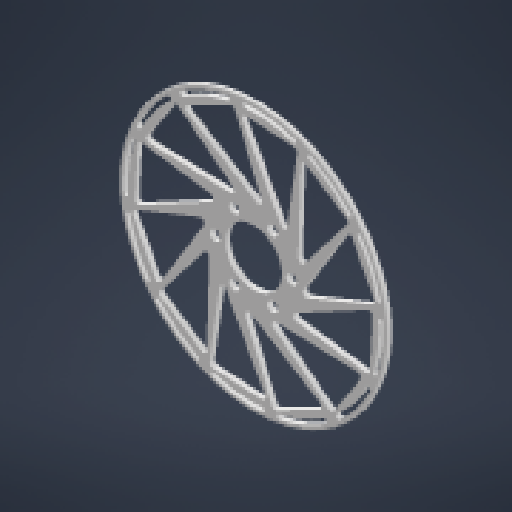
# Autodesk Inventor part: DisqueFrein
Saved by Autodesk Inventor 2026.2 (Build 302298010, 298A)
## iProperties
Created: 2026-04-18
Part Number: DisqueFrein
Material: Générique
Document SubType Name: Modeling
Designer: romai
Density: 1 g/cm^3
Appearance: Par défaut
Author: romai
Autodesk Inventor part; units mm, degrees
ref_plane "YZ Plane" through (0, 0, 0) normal (1, 0, 0) x (0, 1, 0)
ref_plane "XZ Plane" through (0, 0, 0) normal (0, 1, 0) x (-1, 0, 0)
ref_plane "XY Plane" through (0, 0, 0) normal (0, 0, 1) x (1, 0, 0)
sketch "Esquisse1" plane through (0, 0, 0) normal (0, 0, 1) x (1, 0, 0)
  circle A0 centre (0, 0) radius 16.25
  circle A1 centre (0, 0) radius 77.5
  line L0 (1.7183, 28.683) -> (-38.4934, 53.5132)
  line L1 (-10.6387, 68.5856) -> (4.6212, 31.1395)
  arc A2 (1.7183, 28.683) -> (4.6212, 31.1395) centre (2.7691, 30.3848) ccw
  arc A3 (-38.5051, 56.9093) -> (-38.4934, 53.5132) centre (-37.4426, 55.2149) ccw
  arc A4 (-10.6387, 68.5856) -> (-13.2718, 69.672) centre (-12.4908, 67.8308) ccw
  line L2 (-38.5051, 56.9093) -> (-13.2718, 69.672)
  arc A5 (-14.9639, 73.4921) -> (-41.9265, 62.1866) centre (0, 0) ccw
  arc A6 (-14.4371, 71.048) -> (-40.4825, 60.1449) centre (0, 0) ccw
  line L3 (-41.8018, 60.3256) -> (-42.1283, 60.7085)
  line L4 (-13.6695, 72.2839) -> (-13.7977, 72.768)
  arc A7 (-41.8018, 60.3256) -> (-40.4825, 60.1449) centre (-41.0409, 60.9745) ccw
  arc A8 (-41.9265, 62.1866) -> (-42.1283, 60.7085) centre (-41.3675, 61.3574) ccw
  arc A9 (-13.7977, 72.768) -> (-14.9639, 73.4921) centre (-14.7644, 72.5122) ccw
  arc A10 (-14.4371, 71.048) -> (-13.6695, 72.2839) centre (-14.6362, 72.028) ccw
  line L5 (-12.8535, 25.6994) -> (-60.0929, 27.097)
  arc A11 (-61.8011, 30.0323) -> (-60.0929, 27.097) centre (-60.0337, 29.0962) ccw
  line L6 (-61.8011, 30.0323) -> (-46.3297, 53.7019)
  arc A12 (-48.0269, 54.3108) -> (-65.1314, 31.8458) centre (0, 0) ccw
  arc A13 (-66.3642, 31.3426) -> (-65.1314, 31.8458) centre (-66.0297, 32.285) ccw
  arc A14 (-67.4027, 32.8919) -> (-66.8384, 31.5109) centre (-66.504, 32.4533) ccw
  arc A15 (-49.7051, 56.164) -> (-67.4027, 32.8919) centre (0, 0) ccw
  line L7 (-66.3642, 31.3426) -> (-66.8384, 31.5109)
  arc A16 (-48.3331, 56.1201) -> (-49.7051, 56.164) centre (-49.0424, 55.4152) ccw
  line L8 (-47.9801, 55.7649) -> (-48.3331, 56.1201)
  arc A17 (-48.0269, 54.3108) -> (-47.9801, 55.7649) centre (-48.6893, 55.06) ccw
  line L9 (-43.5062, 54.0775) -> (-11.5677, 29.2782)
  arc A18 (-43.5062, 54.0775) -> (-46.3297, 53.7019) centre (-44.7328, 52.4978) ccw
  arc A19 (-12.8535, 25.6994) -> (-11.5677, 29.2782) centre (-12.7943, 27.6985) ccw
  line L10 (-23.9811, 15.8296) -> (-65.5905, -6.5797)
  arc A20 (-68.5375, -4.8918) -> (-65.5905, -6.5797) centre (-66.5388, -4.8188) ccw
  line L11 (-68.5375, -4.8918) -> (-66.9737, 23.3423)
  arc A21 (-68.7479, 23.0211) -> (-72.3283, -4.9864) centre (0, 0) ccw
  arc A22 (-73.1444, -6.0386) -> (-72.3283, -4.9864) centre (-73.3259, -5.0552) ccw
  arc A23 (-74.8184, -5.2162) -> (-73.6392, -6.13) centre (-73.8208, -5.1466) ccw
  arc A24 (-71.1279, 23.7869) -> (-74.8184, -5.2162) centre (0, 0) ccw
  line L12 (-73.1444, -6.0386) -> (-73.6392, -6.13)
  arc A25 (-69.9178, 24.4349) -> (-71.1279, 23.7869) centre (-70.1796, 23.4698) ccw
  line L13 (-69.4344, 24.3038) -> (-69.9178, 24.4349)
  arc A26 (-68.7479, 23.0211) -> (-69.4344, 24.3038) centre (-69.6962, 23.3387) ccw
  line L14 (-64.7162, 25.0794) -> (-24.657, 19.5718)
  arc A27 (-64.7162, 25.0794) -> (-66.9737, 23.3423) centre (-64.9886, 23.098) ccw
  arc A28 (-23.9811, 15.8296) -> (-24.657, 19.5718) centre (-24.9295, 17.5905) ccw
  line L15 (-28.683, 1.7183) -> (-53.5132, -38.4934)
  arc A29 (-56.9093, -38.5051) -> (-53.5132, -38.4934) centre (-55.2149, -37.4426) ccw
  line L16 (-56.9093, -38.5051) -> (-69.672, -13.2718)
  arc A30 (-71.048, -14.4371) -> (-60.1449, -40.4825) centre (0, 0) ccw
  arc A31 (-60.3256, -41.8018) -> (-60.1449, -40.4825) centre (-60.9745, -41.0409) ccw
  arc A32 (-62.1866, -41.9265) -> (-60.7085, -42.1283) centre (-61.3574, -41.3675) ccw
  arc A33 (-73.4921, -14.9639) -> (-62.1866, -41.9265) centre (0, 0) ccw
  line L17 (-60.3256, -41.8018) -> (-60.7085, -42.1283)
  arc A34 (-72.768, -13.7977) -> (-73.4921, -14.9639) centre (-72.5122, -14.7644) ccw
  line L18 (-72.2839, -13.6695) -> (-72.768, -13.7977)
  arc A35 (-71.048, -14.4371) -> (-72.2839, -13.6695) centre (-72.028, -14.6362) ccw
  line L19 (-68.5856, -10.6387) -> (-31.1395, 4.6212)
  arc A36 (-68.5856, -10.6387) -> (-69.672, -13.2718) centre (-67.8308, -12.4908) ccw
  arc A37 (-28.683, 1.7183) -> (-31.1395, 4.6212) centre (-30.3848, 2.7691) ccw
  line L20 (-25.6994, -12.8535) -> (-27.097, -60.0929)
  arc A38 (-30.0323, -61.8011) -> (-27.097, -60.0929) centre (-29.0962, -60.0337) ccw
  line L21 (-30.0323, -61.8011) -> (-53.7019, -46.3297)
  arc A39 (-54.3108, -48.0269) -> (-31.8458, -65.1314) centre (0, 0) ccw
  arc A40 (-31.3426, -66.3642) -> (-31.8458, -65.1314) centre (-32.285, -66.0297) ccw
  arc A41 (-32.8919, -67.4027) -> (-31.5109, -66.8384) centre (-32.4533, -66.504) ccw
  arc A42 (-56.164, -49.7051) -> (-32.8919, -67.4027) centre (0, 0) ccw
  line L22 (-31.3426, -66.3642) -> (-31.5109, -66.8384)
  arc A43 (-56.1201, -48.3331) -> (-56.164, -49.7051) centre (-55.4152, -49.0424) ccw
  line L23 (-55.7649, -47.9801) -> (-56.1201, -48.3331)
  arc A44 (-54.3108, -48.0269) -> (-55.7649, -47.9801) centre (-55.06, -48.6893) ccw
  line L24 (-54.0775, -43.5062) -> (-29.2782, -11.5677)
  arc A45 (-54.0775, -43.5062) -> (-53.7019, -46.3297) centre (-52.4978, -44.7328) ccw
  arc A46 (-25.6994, -12.8535) -> (-29.2782, -11.5677) centre (-27.6985, -12.7943) ccw
  line L25 (-15.8296, -23.9811) -> (6.5797, -65.5905)
  arc A47 (4.8918, -68.5375) -> (6.5797, -65.5905) centre (4.8188, -66.5388) ccw
  line L26 (4.8918, -68.5375) -> (-23.3423, -66.9737)
  arc A48 (-23.0211, -68.7479) -> (4.9864, -72.3283) centre (0, 0) ccw
  arc A49 (6.0386, -73.1444) -> (4.9864, -72.3283) centre (5.0552, -73.3259) ccw
  arc A50 (5.2162, -74.8184) -> (6.13, -73.6392) centre (5.1466, -73.8208) ccw
  arc A51 (-23.7869, -71.1279) -> (5.2162, -74.8184) centre (0, 0) ccw
  line L27 (6.0386, -73.1444) -> (6.13, -73.6392)
  arc A52 (-24.4349, -69.9178) -> (-23.7869, -71.1279) centre (-23.4698, -70.1796) ccw
  line L28 (-24.3038, -69.4344) -> (-24.4349, -69.9178)
  arc A53 (-23.0211, -68.7479) -> (-24.3038, -69.4344) centre (-23.3387, -69.6962) ccw
  line L29 (-25.0794, -64.7162) -> (-19.5718, -24.657)
  arc A54 (-25.0794, -64.7162) -> (-23.3423, -66.9737) centre (-23.098, -64.9886) ccw
  arc A55 (-15.8296, -23.9811) -> (-19.5718, -24.657) centre (-17.5905, -24.9295) ccw
  line L30 (-1.7183, -28.683) -> (38.4934, -53.5132)
  arc A56 (38.5051, -56.9093) -> (38.4934, -53.5132) centre (37.4426, -55.2149) ccw
  line L31 (38.5051, -56.9093) -> (13.2718, -69.672)
  arc A57 (14.4371, -71.048) -> (40.4825, -60.1449) centre (0, 0) ccw
  arc A58 (41.8018, -60.3256) -> (40.4825, -60.1449) centre (41.0409, -60.9745) ccw
  arc A59 (41.9265, -62.1866) -> (42.1283, -60.7085) centre (41.3675, -61.3574) ccw
  arc A60 (14.9639, -73.4921) -> (41.9265, -62.1866) centre (0, 0) ccw
  line L32 (41.8018, -60.3256) -> (42.1283, -60.7085)
  arc A61 (13.7977, -72.768) -> (14.9639, -73.4921) centre (14.7644, -72.5122) ccw
  line L33 (13.6695, -72.2839) -> (13.7977, -72.768)
  arc A62 (14.4371, -71.048) -> (13.6695, -72.2839) centre (14.6362, -72.028) ccw
  line L34 (10.6387, -68.5856) -> (-4.6212, -31.1395)
  arc A63 (10.6387, -68.5856) -> (13.2718, -69.672) centre (12.4908, -67.8308) ccw
  arc A64 (-1.7183, -28.683) -> (-4.6212, -31.1395) centre (-2.7691, -30.3848) ccw
  line L35 (12.8535, -25.6994) -> (60.0929, -27.097)
  arc A65 (61.8011, -30.0323) -> (60.0929, -27.097) centre (60.0337, -29.0962) ccw
  line L36 (61.8011, -30.0323) -> (46.3297, -53.7019)
  arc A66 (48.0269, -54.3108) -> (65.1314, -31.8458) centre (0, 0) ccw
  arc A67 (66.3642, -31.3426) -> (65.1314, -31.8458) centre (66.0297, -32.285) ccw
  arc A68 (67.4027, -32.8919) -> (66.8384, -31.5109) centre (66.504, -32.4533) ccw
  arc A69 (49.7051, -56.164) -> (67.4027, -32.8919) centre (0, 0) ccw
  line L37 (66.3642, -31.3426) -> (66.8384, -31.5109)
  arc A70 (48.3331, -56.1201) -> (49.7051, -56.164) centre (49.0424, -55.4152) ccw
  line L38 (47.9801, -55.7649) -> (48.3331, -56.1201)
  arc A71 (48.0269, -54.3108) -> (47.9801, -55.7649) centre (48.6893, -55.06) ccw
  line L39 (43.5062, -54.0775) -> (11.5677, -29.2782)
  arc A72 (43.5062, -54.0775) -> (46.3297, -53.7019) centre (44.7328, -52.4978) ccw
  arc A73 (12.8535, -25.6994) -> (11.5677, -29.2782) centre (12.7943, -27.6985) ccw
  line L40 (23.9811, -15.8296) -> (65.5905, 6.5797)
  arc A74 (68.5375, 4.8918) -> (65.5905, 6.5797) centre (66.5388, 4.8188) ccw
  line L41 (68.5375, 4.8918) -> (66.9737, -23.3423)
  arc A75 (68.7479, -23.0211) -> (72.3283, 4.9864) centre (0, 0) ccw
  arc A76 (73.1444, 6.0386) -> (72.3283, 4.9864) centre (73.3259, 5.0552) ccw
  arc A77 (74.8184, 5.2162) -> (73.6392, 6.13) centre (73.8208, 5.1466) ccw
  arc A78 (71.1279, -23.7869) -> (74.8184, 5.2162) centre (0, 0) ccw
  line L42 (73.1444, 6.0386) -> (73.6392, 6.13)
  arc A79 (69.9178, -24.4349) -> (71.1279, -23.7869) centre (70.1796, -23.4698) ccw
  line L43 (69.4344, -24.3038) -> (69.9178, -24.4349)
  arc A80 (68.7479, -23.0211) -> (69.4344, -24.3038) centre (69.6962, -23.3387) ccw
  line L44 (64.7162, -25.0794) -> (24.657, -19.5718)
  arc A81 (64.7162, -25.0794) -> (66.9737, -23.3423) centre (64.9886, -23.098) ccw
  arc A82 (23.9811, -15.8296) -> (24.657, -19.5718) centre (24.9295, -17.5905) ccw
  line L45 (28.683, -1.7183) -> (53.5132, 38.4934)
  arc A83 (56.9093, 38.5051) -> (53.5132, 38.4934) centre (55.2149, 37.4426) ccw
  line L46 (56.9093, 38.5051) -> (69.672, 13.2718)
  arc A84 (71.048, 14.4371) -> (60.1449, 40.4825) centre (0, 0) ccw
  arc A85 (60.3256, 41.8018) -> (60.1449, 40.4825) centre (60.9745, 41.0409) ccw
  arc A86 (62.1866, 41.9265) -> (60.7085, 42.1283) centre (61.3574, 41.3675) ccw
  arc A87 (73.4921, 14.9639) -> (62.1866, 41.9265) centre (0, 0) ccw
  line L47 (60.3256, 41.8018) -> (60.7085, 42.1283)
  arc A88 (72.768, 13.7977) -> (73.4921, 14.9639) centre (72.5122, 14.7644) ccw
  line L48 (72.2839, 13.6695) -> (72.768, 13.7977)
  arc A89 (71.048, 14.4371) -> (72.2839, 13.6695) centre (72.028, 14.6362) ccw
  line L49 (68.5856, 10.6387) -> (31.1395, -4.6212)
  arc A90 (68.5856, 10.6387) -> (69.672, 13.2718) centre (67.8308, 12.4908) ccw
  arc A91 (28.683, -1.7183) -> (31.1395, -4.6212) centre (30.3848, -2.7691) ccw
  line L50 (25.6994, 12.8535) -> (27.097, 60.0929)
  arc A92 (30.0323, 61.8011) -> (27.097, 60.0929) centre (29.0962, 60.0337) ccw
  line L51 (30.0323, 61.8011) -> (53.7019, 46.3297)
  arc A93 (54.3108, 48.0269) -> (31.8458, 65.1314) centre (0, 0) ccw
  arc A94 (31.3426, 66.3642) -> (31.8458, 65.1314) centre (32.285, 66.0297) ccw
  arc A95 (32.8919, 67.4027) -> (31.5109, 66.8384) centre (32.4533, 66.504) ccw
  arc A96 (56.164, 49.7051) -> (32.8919, 67.4027) centre (0, 0) ccw
  line L52 (31.3426, 66.3642) -> (31.5109, 66.8384)
  arc A97 (56.1201, 48.3331) -> (56.164, 49.7051) centre (55.4152, 49.0424) ccw
  line L53 (55.7649, 47.9801) -> (56.1201, 48.3331)
  arc A98 (54.3108, 48.0269) -> (55.7649, 47.9801) centre (55.06, 48.6893) ccw
  line L54 (54.0775, 43.5062) -> (29.2782, 11.5677)
  arc A99 (54.0775, 43.5062) -> (53.7019, 46.3297) centre (52.4978, 44.7328) ccw
  arc A100 (25.6994, 12.8535) -> (29.2782, 11.5677) centre (27.6985, 12.7943) ccw
  line L55 (15.8296, 23.9811) -> (-6.5797, 65.5905)
  arc A101 (-4.8918, 68.5375) -> (-6.5797, 65.5905) centre (-4.8188, 66.5388) ccw
  line L56 (-4.8918, 68.5375) -> (23.3423, 66.9737)
  arc A102 (23.0211, 68.7479) -> (-4.9864, 72.3283) centre (0, 0) ccw
  arc A103 (-6.0386, 73.1444) -> (-4.9864, 72.3283) centre (-5.0552, 73.3259) ccw
  arc A104 (-5.2162, 74.8184) -> (-6.13, 73.6392) centre (-5.1466, 73.8208) ccw
  arc A105 (23.7869, 71.1279) -> (-5.2162, 74.8184) centre (0, 0) ccw
  line L57 (-6.0386, 73.1444) -> (-6.13, 73.6392)
  arc A106 (24.4349, 69.9178) -> (23.7869, 71.1279) centre (23.4698, 70.1796) ccw
  line L58 (24.3038, 69.4344) -> (24.4349, 69.9178)
  arc A107 (23.0211, 68.7479) -> (24.3038, 69.4344) centre (23.3387, 69.6962) ccw
  line L59 (25.0794, 64.7162) -> (19.5718, 24.657)
  arc A108 (25.0794, 64.7162) -> (23.3423, 66.9737) centre (23.098, 64.9886) ccw
  arc A109 (15.8296, 23.9811) -> (19.5718, 24.657) centre (17.5905, 24.9295) ccw
  point P0 (-42.8496, 61.5541)
  point P1 (-14.0376, 73.6746)
  point P2 (-41.2192, 59.6425)
  point P3 (-13.3963, 71.2516)
  point P4 (-65.5181, 31.0424)
  point P5 (-47.2273, 55.0076)
  point P6 (-72.2615, -5.8756)
  point P7 (-68.4038, 24.0243)
  point P8 (-59.6425, -41.2192)
  point P9 (-71.2516, -13.3963)
  point P10 (-31.0424, -65.5181)
  point P11 (-55.0076, -47.2273)
  point P12 (5.8756, -72.2615)
  point P13 (-24.0243, -68.4038)
  point P14 (41.2192, -59.6425)
  point P15 (13.3963, -71.2516)
  point P16 (65.5181, -31.0424)
  point P17 (47.2273, -55.0076)
  point P18 (72.2615, 5.8756)
  point P19 (68.4038, -24.0243)
  point P20 (59.6425, 41.2192)
  point P21 (71.2516, 13.3963)
  point P22 (31.0424, 65.5181)
  point P23 (55.0076, 47.2273)
  point P24 (-5.8756, 72.2615)
  point P25 (24.0243, 68.4038)
  dimension "d0" = 32.5
  dimension "d1" = 155
  dimension "d4" = 2
  dimension "d5" = 2
  dimension "d13" = 150
  dimension "d14" = 145
  dimension "d15" = 1
  dimension "d18" = 360
  constraints: 242 point on circle, 120 end point, 110 centre point, 50 point on line, 14 coincident, 12 tangent, 4 equal radius, 469 other
  measures "d0" diameter of A0
  measures "d1" diameter of A1
  measures "d4" radius of A2
  measures "d5" radius of A4
  measures "d13" diameter of A5
  measures "d14" diameter of A6
  measures "d15" radius of A7
extrude "Extrusion1" add sketch "Esquisse1" along normal blind 3
fillet "Congé1" radius 1 2 edges at (-77.5, 0, 3) (-77.5, 0, 0)
sketch "Esquisse2" plane through (0, 0, 3) normal (0, 0, 1) x (1, 0, 0)
  circle A0 centre (0, 0) radius 22
  line L0 (0, 0) -> (22, 0)
  dimension "d28" = 44
  constraints: 2 end point, 1 coincident, 1 horizontal, 1 horizontal alignment, 2 other
hole "Perçage1" at (22, 0, 3) direction (0, 0, -1) diameter 5.917 end through all
pattern_circular "Réseau circulaire1" count 6 over 360 about axis through (0, 0, 0) along (0, 0, 1) of "Perçage1"
